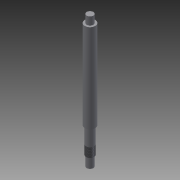
# Autodesk Inventor part: 1605_400mm
Saved by Autodesk Inventor 2014 (Build 180170000, 170)
## iProperties
Created: 2014-08-11
Part Number: 1605_400mm
Material: Generic
Document SubType Name: Modeling
Designer: Matthew
Density: 1 g/cm^3
Appearance: Default
Author: Matthew
Autodesk Inventor part; units mm, degrees
ref_plane "YZ Plane" through (0, 0, 0) normal (1, 0, 0) x (0, 1, 0)
ref_plane "XZ Plane" through (0, 0, 0) normal (0, 1, 0) x (-1, 0, 0)
ref_plane "XY Plane" through (0, 0, 0) normal (0, 0, 1) x (1, 0, 0)
sketch "Sketch1" plane through (0, 0, 0) normal (0, 1, 0) x (-1, 0, 0)
  circle A0 centre (0, 0) radius 8
  dimension "d0" = 16
  constraints: 1 centre point, 1 coincident
  measures "d0" diameter of A0
extrude "Extrusion1" add sketch "Sketch1" along normal blind 200
sketch "Sketch2" plane through (0, 0, 0) normal (0, -1, 0) x (1, 0, 0)
  circle A0 centre (0, 0) radius 8 projected
extrude "Extrusion2" cut sketch "Sketch2" against normal blind 50
sketch "Sketch3" plane through (0, 50, 0) normal (0, -1, 0) x (1, 0, 0)
  circle A0 centre (0, 0) radius 8 projected
extrude "Extrusion3" add sketch "Sketch3" along normal blind 50
sketch "Sketch4" plane through (0, 0, 0) normal (0, -1, 0) x (1, 0, 0)
  circle A0 centre (0, 0) radius 8 projected
  circle A1 centre (0, 0) radius 6
  dimension "d7" = 12
  constraints: 1 centre point, 1 coincident
  measures "d7" diameter of A1
extrude "Extrusion4" cut sketch "Sketch4" against normal blind 14
thread "Thread1" size "M12x1" class "6g" standard "ANSI Metric M Profile" full length
sketch "Sketch6" plane through (0, 14, 0) normal (0, -1, 0) x (1, 0, 0)
  circle A0 centre (0, 0) radius 8 projected
  circle A1 centre (0, 0) radius 6.05
  dimension "d13" = 12.1
  constraints: 1 centre point, 1 coincident
  measures "d13" diameter of A1
extrude "Extrusion5" cut sketch "Sketch6" against normal blind 25
sketch "Sketch7" plane through (0, 0, 0) normal (0, -1, 0) x (1, 0, 0)
  circle A0 centre (0, 0) radius 6 projected
  circle A1 centre (0, 0) radius 5
  dimension "d16" = 10
  constraints: 1 centre point, 1 coincident
  measures "d16" diameter of A1
extrude "Extrusion6" add sketch "Sketch7" along normal blind 15 contours A1
sketch "Sketch8" plane through (0, 200, 0) normal (0, 1, 0) x (1, 0, 0)
  circle A0 centre (0, 0) radius 8 projected
extrude "Extrusion7" cut sketch "Sketch8" against normal blind 27.101
sketch "Sketch9" plane through (0, 172.899, 0) normal (0, 1, 0) x (1, 0, 0)
  circle A0 centre (0, 0) radius 8 projected
  circle A1 centre (0, 0) radius 5
  dimension "d21" = 10
  constraints: 1 centre point, 1 coincident
  measures "d21" diameter of A1
extrude "Extrusion8" add sketch "Sketch9" along normal blind 12 contours A1
body "Solid1"
